Autodesk Inventor part; units mm, degrees
(part 2 of 2)
sketch "Sketch12" plane through (0, 0, 3) normal (0, 0, 1) x (1, 0, 0)
  circle A0 centre (14, 34.5) radius 1.5 projected
  circle A1 centre (-40, -22.5) radius 1.5 projected
  circle A2 centre (-40, 35.5) radius 1.5 projected
  circle A3 centre (46, -22.5) radius 1.5 projected
  circle A4 centre (46, 35.5) radius 1.5 projected
  arc A5 (42.6, 39.5) -> (42, 38.9) centre (42.6, 38.9) ccw projected
  line L0 (42, 38.9) -> (42, 11.25) projected
  arc A6 (40.25, 9.5) -> (42, 11.25) centre (40.25, 11.25) ccw projected
  line L1 (40.25, 9.5) -> (25.75, 9.5) projected
  arc A7 (24, 11.25) -> (25.75, 9.5) centre (25.75, 11.25) ccw projected
  line L2 (24, 11.25) -> (24, 38.9) projected
  arc A8 (24, 38.9) -> (23.4, 39.5) centre (23.4, 38.9) ccw projected
  line L3 (23.4, 39.5) -> (-49.4, 39.5) projected
  arc A9 (-49.4, 39.5) -> (-50, 38.9) centre (-49.4, 38.9) ccw projected
  line L4 (-50, 38.9) -> (-50, 14.5) projected
  line L5 (-78, 14.5) -> (-50, 14.5) projected
  line L6 (-78, -39.5) -> (-78, 14.5) projected
  line L7 (-78, -39.5) -> (49.4, -39.5) projected
  arc A10 (49.4, -39.5) -> (50, -38.9) centre (49.4, -38.9) ccw projected
  line L8 (50, -38.9) -> (50, 38.9) projected
  arc A11 (50, 38.9) -> (49.4, 39.5) centre (49.4, 38.9) ccw projected
  line L9 (49.4, 39.5) -> (42.6, 39.5) projected
  line L10 (-28.5547, -12.5) -> (-27.0547, -12.5) projected
  arc A12 (-25.3047, -14.25) -> (-27.0547, -12.5) centre (-27.0547, -14.25) ccw projected
  line L11 (-25.3047, -14.25) -> (-25.3047, -14.75) projected
  arc A13 (-27.0547, -16.5) -> (-25.3047, -14.75) centre (-27.0547, -14.75) ccw projected
  line L12 (-27.0547, -16.5) -> (-28.5547, -16.5) projected
  arc A14 (-30.3047, -14.75) -> (-28.5547, -16.5) centre (-28.5547, -14.75) ccw projected
  line L13 (-30.3047, -14.75) -> (-30.3047, -14.25) projected
  arc A15 (-28.5547, -12.5) -> (-30.3047, -14.25) centre (-28.5547, -14.25) ccw projected
  line L14 (2.5, -14.25) -> (2.5, -14.75) projected
  arc A16 (0.75, -16.5) -> (2.5, -14.75) centre (0.75, -14.75) ccw projected
  line L15 (0.75, -16.5) -> (-0.75, -16.5) projected
  arc A17 (-2.5, -14.75) -> (-0.75, -16.5) centre (-0.75, -14.75) ccw projected
  line L16 (-2.5, -14.75) -> (-2.5, -14.25) projected
  arc A18 (-0.75, -12.5) -> (-2.5, -14.25) centre (-0.75, -14.25) ccw projected
  line L17 (-0.75, -12.5) -> (0.75, -12.5) projected
  arc A19 (2.5, -14.25) -> (0.75, -12.5) centre (0.75, -14.25) ccw projected
  line L18 (37.5, -14.75) -> (37.5, -14.25) projected
  arc A20 (39.25, -12.5) -> (37.5, -14.25) centre (39.25, -14.25) ccw projected
  line L19 (39.25, -12.5) -> (40.75, -12.5) projected
  arc A21 (42.5, -14.25) -> (40.75, -12.5) centre (40.75, -14.25) ccw projected
  line L20 (42.5, -14.25) -> (42.5, -14.75) projected
  arc A22 (40.75, -16.5) -> (42.5, -14.75) centre (40.75, -14.75) ccw projected
  line L21 (40.75, -16.5) -> (39.25, -16.5) projected
  arc A23 (37.5, -14.75) -> (39.25, -16.5) centre (39.25, -14.75) ccw projected
  line L22 (32.75, -27) -> (33.25, -27) projected
  arc A24 (35, -28.75) -> (33.25, -27) centre (33.25, -28.75) ccw projected
  line L23 (35, -28.75) -> (35, -30.25) projected
  arc A25 (33.25, -32) -> (35, -30.25) centre (33.25, -30.25) ccw projected
  line L24 (33.25, -32) -> (32.75, -32) projected
  arc A26 (31, -30.25) -> (32.75, -32) centre (32.75, -30.25) ccw projected
  line L25 (31, -30.25) -> (31, -28.75) projected
  arc A27 (32.75, -27) -> (31, -28.75) centre (32.75, -28.75) ccw projected
  line L26 (-2.5, 18.75) -> (-2.5, 20.25) projected
  arc A28 (-0.75, 22) -> (-2.5, 20.25) centre (-0.75, 20.25) ccw projected
  line L27 (-0.75, 22) -> (-0.25, 22) projected
  arc A29 (1.5, 20.25) -> (-0.25, 22) centre (-0.25, 20.25) ccw projected
  line L28 (1.5, 20.25) -> (1.5, 18.75) projected
  arc A30 (-0.25, 17) -> (1.5, 18.75) centre (-0.25, 18.75) ccw projected
  line L29 (-0.25, 17) -> (-0.75, 17) projected
  arc A31 (-2.5, 18.75) -> (-0.75, 17) centre (-0.75, 18.75) ccw projected
  line L30 (-30.3047, 5.25) -> (-30.3047, 5.75) projected
  arc A32 (-28.5547, 7.5) -> (-30.3047, 5.75) centre (-28.5547, 5.75) ccw projected
  line L31 (-28.5547, 7.5) -> (-27.0547, 7.5) projected
  arc A33 (-25.3047, 5.75) -> (-27.0547, 7.5) centre (-27.0547, 5.75) ccw projected
  line L32 (-25.3047, 5.75) -> (-25.3047, 5.25) projected
  arc A34 (-27.0547, 3.5) -> (-25.3047, 5.25) centre (-27.0547, 5.25) ccw projected
  line L33 (-27.0547, 3.5) -> (-28.5547, 3.5) projected
  arc A35 (-30.3047, 5.25) -> (-28.5547, 3.5) centre (-28.5547, 5.25) ccw projected
  line L34 (-0.75, -26.5) -> (0.75, -26.5) projected
  arc A36 (2.5, -28.25) -> (0.75, -26.5) centre (0.75, -28.25) ccw projected
  line L35 (2.5, -28.25) -> (2.5, -28.75) projected
  arc A37 (0.75, -30.5) -> (2.5, -28.75) centre (0.75, -28.75) ccw projected
  line L36 (0.75, -30.5) -> (-0.75, -30.5) projected
  arc A38 (-2.5, -28.75) -> (-0.75, -30.5) centre (-0.75, -28.75) ccw projected
  line L37 (-2.5, -28.75) -> (-2.5, -28.25) projected
  arc A39 (-0.75, -26.5) -> (-2.5, -28.25) centre (-0.75, -28.25) ccw projected
  line L38 (39.25, 7.5) -> (40.75, 7.5) projected
  arc A40 (42.5, 5.75) -> (40.75, 7.5) centre (40.75, 5.75) ccw projected
  line L39 (42.5, 5.75) -> (42.5, 5.25) projected
  arc A41 (40.75, 3.5) -> (42.5, 5.25) centre (40.75, 5.25) ccw projected
  line L40 (40.75, 3.5) -> (39.25, 3.5) projected
  arc A42 (37.5, 5.25) -> (39.25, 3.5) centre (39.25, 5.25) ccw projected
  line L41 (37.5, 5.25) -> (37.5, 5.75) projected
  arc A43 (39.25, 7.5) -> (37.5, 5.75) centre (39.25, 5.75) ccw projected
  line L42 (19.25, -32) -> (18.75, -32) projected
  arc A44 (17, -30.25) -> (18.75, -32) centre (18.75, -30.25) ccw projected
  line L43 (17, -30.25) -> (17, -28.75) projected
  arc A45 (18.75, -27) -> (17, -28.75) centre (18.75, -28.75) ccw projected
  line L44 (18.75, -27) -> (19.25, -27) projected
  arc A46 (21, -28.75) -> (19.25, -27) centre (19.25, -28.75) ccw projected
  line L45 (21, -28.75) -> (21, -30.25) projected
  arc A47 (19.25, -32) -> (21, -30.25) centre (19.25, -30.25) ccw projected
  line L46 (-22.5, 18.75) -> (-22.5, 20.25) projected
  arc A48 (-20.75, 22) -> (-22.5, 20.25) centre (-20.75, 20.25) ccw projected
  line L47 (-20.75, 22) -> (-20.25, 22) projected
  arc A49 (-18.5, 20.25) -> (-20.25, 22) centre (-20.25, 20.25) ccw projected
  line L48 (-18.5, 20.25) -> (-18.5, 18.75) projected
  arc A50 (-20.25, 17) -> (-18.5, 18.75) centre (-20.25, 18.75) ccw projected
  line L49 (-20.25, 17) -> (-20.75, 17) projected
  arc A51 (-22.5, 18.75) -> (-20.75, 17) centre (-20.75, 18.75) ccw projected
  line L50 (-24, -34.25) -> (-24, -32.75) projected
  arc A52 (-22.25, -31) -> (-24, -32.75) centre (-22.25, -32.75) ccw projected
  line L51 (-22.25, -31) -> (-21.75, -31) projected
  arc A53 (-20, -32.75) -> (-21.75, -31) centre (-21.75, -32.75) ccw projected
  line L52 (-20, -32.75) -> (-20, -34.25) projected
  arc A54 (-21.75, -36) -> (-20, -34.25) centre (-21.75, -34.25) ccw projected
  line L53 (-21.75, -36) -> (-22.25, -36) projected
  arc A55 (-24, -34.25) -> (-22.25, -36) centre (-22.25, -34.25) ccw projected
  line L54 (40.2277, -23) -> (39.7277, -23) projected
  arc A56 (37.9777, -21.25) -> (39.7277, -23) centre (39.7277, -21.25) ccw projected
  line L55 (37.9777, -21.25) -> (37.9777, -19.75) projected
  arc A57 (39.7277, -18) -> (37.9777, -19.75) centre (39.7277, -19.75) ccw projected
  line L56 (39.7277, -18) -> (40.2277, -18) projected
  arc A58 (41.9777, -19.75) -> (40.2277, -18) centre (40.2277, -19.75) ccw projected
  line L57 (41.9777, -19.75) -> (41.9777, -21.25) projected
  arc A59 (40.2277, -23) -> (41.9777, -21.25) centre (40.2277, -21.25) ccw projected
  line L58 (-33, -34.25) -> (-33, -32.75) projected
  arc A60 (-31.25, -31) -> (-33, -32.75) centre (-31.25, -32.75) ccw projected
  line L59 (-31.25, -31) -> (-30.75, -31) projected
  arc A61 (-29, -32.75) -> (-30.75, -31) centre (-30.75, -32.75) ccw projected
  line L60 (-29, -32.75) -> (-29, -34.25) projected
  arc A62 (-30.75, -36) -> (-29, -34.25) centre (-30.75, -34.25) ccw projected
  line L61 (-30.75, -36) -> (-31.25, -36) projected
  arc A63 (-33, -34.25) -> (-31.25, -36) centre (-31.25, -34.25) ccw projected
  line L62 (28.9777, -21.25) -> (28.9777, -19.75) projected
  arc A64 (30.7277, -18) -> (28.9777, -19.75) centre (30.7277, -19.75) ccw projected
  line L63 (30.7277, -18) -> (31.2277, -18) projected
  arc A65 (32.9777, -19.75) -> (31.2277, -18) centre (31.2277, -19.75) ccw projected
  line L64 (32.9777, -19.75) -> (32.9777, -21.25) projected
  arc A66 (31.2277, -23) -> (32.9777, -21.25) centre (31.2277, -21.25) ccw projected
  line L65 (31.2277, -23) -> (30.7277, -23) projected
  arc A67 (28.9777, -21.25) -> (30.7277, -23) centre (30.7277, -21.25) ccw projected
  line L66 (5.75, 11.5) -> (4.25, 11.5) projected
  arc A68 (2.5, 13.25) -> (4.25, 11.5) centre (4.25, 13.25) ccw projected
  line L67 (2.5, 13.25) -> (2.5, 13.75) projected
  arc A69 (4.25, 15.5) -> (2.5, 13.75) centre (4.25, 13.75) ccw projected
  line L68 (4.25, 15.5) -> (5.75, 15.5) projected
  arc A70 (7.5, 13.75) -> (5.75, 15.5) centre (5.75, 13.75) ccw projected
  line L69 (7.5, 13.75) -> (7.5, 13.25) projected
  arc A71 (5.75, 11.5) -> (7.5, 13.25) centre (5.75, 13.25) ccw projected
  line L70 (-32.5, 7.75) -> (-32.5, 7.25) projected
  arc A72 (-34.25, 5.5) -> (-32.5, 7.25) centre (-34.25, 7.25) ccw projected
  line L71 (-34.25, 5.5) -> (-35.75, 5.5) projected
  arc A73 (-37.5, 7.25) -> (-35.75, 5.5) centre (-35.75, 7.25) ccw projected
  line L72 (-37.5, 7.25) -> (-37.5, 7.75) projected
  arc A74 (-35.75, 9.5) -> (-37.5, 7.75) centre (-35.75, 7.75) ccw projected
  line L73 (-35.75, 9.5) -> (-34.25, 9.5) projected
  arc A75 (-32.5, 7.75) -> (-34.25, 9.5) centre (-34.25, 7.75) ccw projected
  line L74 (7.5, 7.75) -> (7.5, 7.25) projected
  arc A76 (5.75, 5.5) -> (7.5, 7.25) centre (5.75, 7.25) ccw projected
  line L75 (5.75, 5.5) -> (4.25, 5.5) projected
  arc A77 (2.5, 7.25) -> (4.25, 5.5) centre (4.25, 7.25) ccw projected
  line L76 (2.5, 7.25) -> (2.5, 7.75) projected
  arc A78 (4.25, 9.5) -> (2.5, 7.75) centre (4.25, 7.75) ccw projected
  line L77 (4.25, 9.5) -> (5.75, 9.5) projected
  arc A79 (7.5, 7.75) -> (5.75, 9.5) centre (5.75, 7.75) ccw projected
  line L78 (-34.25, 11.5) -> (-35.75, 11.5) projected
  arc A80 (-37.5, 13.25) -> (-35.75, 11.5) centre (-35.75, 13.25) ccw projected
  line L79 (-37.5, 13.25) -> (-37.5, 13.75) projected
  arc A81 (-35.75, 15.5) -> (-37.5, 13.75) centre (-35.75, 13.75) ccw projected
  line L80 (-35.75, 15.5) -> (-34.25, 15.5) projected
  arc A82 (-32.5, 13.75) -> (-34.25, 15.5) centre (-34.25, 13.75) ccw projected
  line L81 (-32.5, 13.75) -> (-32.5, 13.25) projected
  arc A83 (-34.25, 11.5) -> (-32.5, 13.25) centre (-34.25, 13.25) ccw projected
  line L82 (-50, 14.5) -> (-78, 14.5)
  line L83 (-78, 14.5) -> (-78, -18.5)
  line L84 (-78, -18.5) -> (-50, -18.5)
  line L85 (-50, -18.5) -> (-50, 14.5)
  line L86 (-78, -39.5) -> (-78, 14.5) projected
  point P0 (0, 0)
  point P1 (-78, -18.5)
  dimension "d163" = 33
  constraints: 8 end point, 2 parallel, 1 horizontal, 1 perpendicular, 1 point on line
  measures "d163" distance between parallel lines of L5 L84
extrude "Extrusion12" cut sketch "Sketch12" against normal blind 4.6 contours L6 L5 L85 L84
fillet "Fillet7" radius 1.75 1 edges at (-50, -18.5, 0.7)
sketch "Sketch13" plane through (0, 0, -1.6) normal (0, 0, 1) x (1, 0, 0)
  arc A0 (-51.75, -18.5) -> (-50, -16.75) centre (-51.75, -16.75) ccw projected
  line L0 (-50, 14.5) -> (-50, -16.75) projected
  line L1 (-78, 14.5) -> (-50, 14.5) projected
  line L2 (-78, -18.5) -> (-78, 14.5) projected
  line L3 (-51.75, -18.5) -> (-78, -18.5) projected
  line L4 (-64, 14.5) -> (-64, -18.5) construction
  circle A1 centre (-64, 11.325) radius 1.75
  circle A2 centre (-64, -14.075) radius 1.75
  point P0 (0, 0)
  dimension "d169" = 3.5
  dimension "d170" = 3.5
  dimension "d171" = 25.4
  dimension "d172" = 3.175
  constraints: 3 point on line, 2 centre point, 2 end point, 1 midpoint, 1 perpendicular
  measures "d169" diameter of A1
  measures "d170" diameter of A2
  measures "d171" distance of A2.centre A1.centre
  measures "d172" distance from line of L1 A1.centre
extrude "Extrusion13" cut sketch "Sketch13" against normal through all contours A1 | A2
sketch "Sketch14" plane through (0, 0, 3) normal (0, 0, 1) x (1, 0, 0)
  line L0 (-78, -39.5) -> (49.4, -39.5) projected
  line L1 (-78, -39.5) -> (-50, -39.5)
  line L2 (-50, -39.5) -> (-50, -29.5)
  line L3 (-50, -29.5) -> (-78, -29.5)
  line L4 (-78, -29.5) -> (-78, -39.5)
  point P0 (0, 0)
  point P1 (-50, -16.75)
  dimension "d175" = 10
  constraints: 8 end point, 2 parallel, 1 horizontal, 1 perpendicular, 1 point on line
  measures "d175" distance between parallel lines of L0 L3
extrude "Extrusion14" cut sketch "Sketch14" against normal through all
fillet "Fillet8" radius 1.75 1 edges at (-50, -29.5, -0.3)
fillet "Fillet9" radius 0.6 4 edges at (-78, 14.5, -2.6) (-78, -18.5, 0.7) (-78, -29.5, -0.3) (-50, -39.5, -0.3)
sketch "Sketch15" plane through (0, 0, -3.6) normal (0, 0, -1) x (-1, 0, 0)
  line L0 (47, -39.5) -> (78, -39.5)
  line L1 (78, -39.5) -> (78, -20.5)
  line L2 (78, -20.5) -> (47, -20.5)
  line L3 (47, -20.5) -> (47, -39.5)
  line L4 (78, -28.9) -> (78, 13.9) projected
  line L5 (51.75, -18.5) -> (77.4, -18.5) projected
  point P0 (0, 0)
  dimension "d180" = 2
  constraints: 8 end point, 2 parallel, 1 horizontal, 1 perpendicular, 1 point on line
  measures "d180" distance between parallel lines of L5 L2
extrude "Extrusion15" cut sketch "Sketch15" against normal up to surface (3.6 mm away)
fillet "Fillet10" radius 0.6 3 edges at (-47, -20.5, -1.8) (-47, 14.5, -1.8) (-78, -20.5, -1.8)
sketch "Sketch16" plane through (0, 0, 3) normal (0, 0, 1) x (1, 0, 0)
  line L0 (-78, -28.9) -> (-78, -19.1) projected
  line L1 (-73.75, -21) -> (-72.25, -21)
  line L2 (-70.5, -22.75) -> (-70.5, -23.25)
  line L3 (-72.25, -25) -> (-73.75, -25)
  line L4 (-75.5, -23.25) -> (-75.5, -22.75)
  line L5 (-75.5, -21) -> (-70.5, -25) construction
  line L6 (-70.5, -21) -> (-75.5, -25) construction
  arc A0 (-70.5, -22.75) -> (-72.25, -21) centre (-72.25, -22.75) ccw
  arc A1 (-72.25, -25) -> (-70.5, -23.25) centre (-72.25, -23.25) ccw
  arc A2 (-75.5, -23.25) -> (-73.75, -25) centre (-73.75, -23.25) ccw
  arc A3 (-73.75, -21) -> (-75.5, -22.75) centre (-73.75, -22.75) ccw
  line L7 (-77.4, -29.5) -> (-51.75, -29.5) projected
  line L8 (-67.386, -26.25) -> (-82.3219, -26.25) construction
  line L9 (-73.75, -31.5) -> (-72.25, -31.5)
  line L10 (-70.5, -29.75) -> (-70.5, -29.25)
  line L11 (-72.25, -27.5) -> (-73.75, -27.5)
  line L12 (-75.5, -29.25) -> (-75.5, -29.75)
  line L13 (-75.5, -31.5) -> (-70.5, -27.5) construction
  line L14 (-70.5, -31.5) -> (-75.5, -27.5) construction
  arc A4 (-72.25, -31.5) -> (-70.5, -29.75) centre (-72.25, -29.75) ccw
  arc A5 (-70.5, -29.25) -> (-72.25, -27.5) centre (-72.25, -29.25) ccw
  arc A6 (-73.75, -27.5) -> (-75.5, -29.25) centre (-73.75, -29.25) ccw
  arc A7 (-75.5, -29.75) -> (-73.75, -31.5) centre (-73.75, -29.75) ccw
  line L15 (-20.75, 37) -> (-21.25, 37)
  line L16 (-23, 35.25) -> (-23, 33.75)
  line L17 (-21.25, 32) -> (-20.75, 32)
  line L18 (-19, 33.75) -> (-19, 35.25)
  line L19 (-19, 37) -> (-23, 32) construction
  line L20 (-23, 37) -> (-19, 32) construction
  line L21 (-27.25, 37) -> (-27.75, 37)
  line L22 (-29.5, 35.25) -> (-29.5, 33.75)
  line L23 (-27.75, 32) -> (-27.25, 32)
  line L24 (-25.5, 33.75) -> (-25.5, 35.25)
  line L25 (-25.5, 37) -> (-29.5, 32) construction
  line L26 (-29.5, 37) -> (-25.5, 32) construction
  arc A8 (-19, 35.25) -> (-20.75, 37) centre (-20.75, 35.25) ccw
  arc A9 (-20.75, 32) -> (-19, 33.75) centre (-20.75, 33.75) ccw
  arc A10 (-23, 33.75) -> (-21.25, 32) centre (-21.25, 33.75) ccw
  arc A11 (-21.25, 37) -> (-23, 35.25) centre (-21.25, 35.25) ccw
  arc A12 (-25.5, 35.25) -> (-27.25, 37) centre (-27.25, 35.25) ccw
  arc A13 (-27.25, 32) -> (-25.5, 33.75) centre (-27.25, 33.75) ccw
  arc A14 (-29.5, 33.75) -> (-27.75, 32) centre (-27.75, 33.75) ccw
  arc A15 (-27.75, 37) -> (-29.5, 35.25) centre (-27.75, 35.25) ccw
  line L27 (-50, 38.9) -> (-50, -16.75) projected
  line L28 (23.4, 39.5) -> (-49.4, 39.5) projected
  point P0 (0, 0)
  point P1 (-73, -23)
  point P2 (-73, -29.5)
  point P3 (-73, -29.5)
  point P4 (-21, 34.5)
  point P5 (-27.5, 34.5)
  dimension "d187" = 1.75
  dimension "d188" = 1.5
  dimension "d189" = 0.5
  dimension "d190" = 5
  dimension "d196" = 2.5
  dimension "d197" = 2.5
  dimension "d198" = 1.75
  dimension "d199" = 0.5
  dimension "d200" = 0.5
  dimension "d201" = 1.5
  dimension "d202" = 1.5
  dimension "d203" = 22.5
  dimension "d204" = 5
  constraints: 50 end point, 34 point on line, 32 point on circle, 24 tangent, 17 symmetric about line, 16 centre point, 10 equal radius, 7 midpoint, 6 parallel, 4 horizontal, 3 perpendicular, 4 other
  measures "d187" radius of A0
  measures "d188" distance of L3.start L3.end
  measures "d189" distance of L2.start L2.end
  measures "d190" distance from line of L0 point (-73, -23)
  measures "d196" distance between parallel lines of L11 L3
  measures "d197" distance between parallel lines of L16 L24
  measures "d198" radius of A8
  measures "d199" distance of L17.start L17.end
  measures "d200" distance of L23.start L23.end
  measures "d201" distance of L24.start L24.end
  measures "d202" distance of L18.start L18.end
  measures "d203" distance from line of L27 point (-27.5, 34.5)
  measures "d204" distance from line of L28 point (-21, 34.5)
extrude "Extrusion16" cut sketch "Sketch16" against normal through all
fillet "Fillet11" radius 0.6 2 edges at (-70.5, -29.5, 1.5) (-75.5, -29.5, 1.5)
chamfer "Chamfer1" distance 0.5 angle 45 198 edges at (-50, 11.075, 3) (-50.5126, -17.9874, 3) (-64.575, -18.5, 3) (-77.8243, -18.6757, 3) (-78, -24, 3) (-77.8243, -29.3243, 3) (-76.7369, -29.5, 3) (-75.6824, -29.3548, 3) (-74.8916, -27.9236, 3) (-73, -27.5, 3) (-71.1084, -27.9236, 3) (-70.3176, -29.3548, 3) (-60.8381, -29.5, 3) (-50.5126, -30.0126, 3) (-50, -35.075, 3) (-49.8243, -39.3243, 3) (0, -39.5, 3) (49.8243, -39.3243, 3) (50, 0, 3) (49.8243, 39.3243, 3) (46, 39.5, 3) (42.1757, 39.3243, 3) (42, 25.075, 3) (41.4874, 10.0126, 3) (33, 9.5, 3) (24.5126, 10.0126, 3) (24, 25.075, 3) (23.8243, 39.3243, 3) (-13, 39.5, 3) (-49.8243, 39.3243, 3) (-19.0126, 21.4874, 3) (-20.5, 22, 3) (-21.9874, 21.4874, 3) (-22.5, 19.5, 3) (-21.9874, 17.5126, 3) (-20.5, 17, 3) (-19.0126, 17.5126, 3) (-18.5, 19.5, 3) (-33.0126, 14.9874, 3) (-35, 15.5, 3) (-36.9874, 14.9874, 3) (-37.5, 13.5, 3) (-36.9874, 12.0126, 3) (-35, 11.5, 3) (-33.0126, 12.0126, 3) (-32.5, 13.5, 3) (-25.8172, 6.9874, 3) (-27.8047, 7.5, 3) (-29.7921, 6.9874, 3) (-30.3047, 5.5, 3) (-29.7921, 4.0126, 3) (-27.8047, 3.5, 3) (-25.8172, 4.0126, 3) (-25.3047, 5.5, 3) (-33.0126, 8.9874, 3) (-35, 9.5, 3) (-36.9874, 8.9874, 3) (-37.5, 7.5, 3) (-36.9874, 6.0126, 3) (-35, 5.5, 3) (-33.0126, 6.0126, 3) (-32.5, 7.5, 3) (-27.8047, -12.5, 3) (-25.8172, -13.0126, 3) (-25.3047, -14.5, 3) (-25.8172, -15.9874, 3) (-27.8047, -16.5, 3) (-29.7921, -15.9874, 3) (-30.3047, -14.5, 3) (-29.7921, -13.0126, 3) (-29.5126, -31.5126, 3) (-31, -31, 3) (-32.4874, -31.5126, 3) (-33, -33.5, 3) (-32.4874, -35.4874, 3) (-31, -36, 3) (-29.5126, -35.4874, 3) (-29, -33.5, 3) (-20.5126, -31.5126, 3) (-22, -31, 3) (-23.4874, -31.5126, 3) (-24, -33.5, 3) (-23.4874, -35.4874, 3) (-22, -36, 3) (-20.5126, -35.4874, 3) (-20, -33.5, 3) (0, -26.5, 3) (1.9874, -27.0126, 3) (2.5, -28.5, 3) (1.9874, -29.9874, 3) (0, -30.5, 3) (-1.9874, -29.9874, 3) (-2.5, -28.5, 3) (-1.9874, -27.0126, 3) (1.9874, -13.0126, 3) (0, -12.5, 3) (-1.9874, -13.0126, 3) (-2.5, -14.5, 3) (-1.9874, -15.9874, 3) (0, -16.5, 3) (1.9874, -15.9874, 3) (2.5, -14.5, 3) (17.5126, -27.5126, 3) (17, -29.5, 3) (17.5126, -31.4874, 3) (19, -32, 3) (20.4874, -31.4874, 3) (21, -29.5, 3) (20.4874, -27.5126, 3) (19, -27, 3) (34.4874, -27.5126, 3) (33, -27, 3) (31.5126, -27.5126, 3) (31, -29.5, 3) (31.5126, -31.4874, 3) (33, -32, 3) (34.4874, -31.4874, 3) (35, -29.5, 3) (32.4652, -18.5126, 3) (30.9777, -18, 3) (29.4903, -18.5126, 3) (28.9777, -20.5, 3) (29.4903, -22.4874, 3) (30.9777, -23, 3) (32.4652, -22.4874, 3) (32.9777, -20.5, 3) (41.9874, -13.0126, 3) (40, -12.5, 3) (38.0126, -13.0126, 3) (37.5, -14.5, 3) (38.0126, -15.9874, 3) (40, -16.5, 3) (41.9874, -15.9874, 3) (42.5, -14.5, 3) (41.4652, -18.5126, 3) (39.9777, -18, 3) (38.4903, -18.5126, 3) (37.9777, -20.5, 3) (38.4903, -22.4874, 3) (39.9777, -23, 3) (41.4652, -22.4874, 3) (41.9777, -20.5, 3) (41.9874, 6.9874, 3) (40, 7.5, 3) (38.0126, 6.9874, 3) (37.5, 5.5, 3) (38.0126, 4.0126, 3) (40, 3.5, 3) (41.9874, 4.0126, 3) (42.5, 5.5, 3) (6.9874, 8.9874, 3) (5, 9.5, 3) (3.0126, 8.9874, 3) (2.5, 7.5, 3) (3.0126, 6.0126, 3) (5, 5.5, 3) (6.9874, 6.0126, 3) (7.5, 7.5, 3) (6.9874, 14.9874, 3) (5, 15.5, 3) (3.0126, 14.9874, 3) (2.5, 13.5, 3) (3.0126, 12.0126, 3) (5, 11.5, 3) (6.9874, 12.0126, 3) (7.5, 13.5, 3) (0.9874, 21.4874, 3) (-0.5, 22, 3) (-1.9874, 21.4874, 3) (-2.5, 19.5, 3) (-1.9874, 17.5126, 3) (-0.5, 17, 3) (0.9874, 17.5126, 3) (1.5, 19.5, 3) (-71.0126, -21.5126, 3) (-70.5, -23, 3) (-71.0126, -24.4874, 3) (-73, -25, 3) (-74.9874, -24.4874, 3) (-75.5, -23, 3) (-74.9874, -21.5126, 3) (-73, -21, 3) (-25.5, 34.5, 3) (-26.0126, 32.5126, 3) (-27.5, 32, 3) (-28.9874, 32.5126, 3) (-29.5, 34.5, 3) (-28.9874, 36.4874, 3) (-27.5, 37, 3) (-26.0126, 36.4874, 3) (-21, 32, 3) (-22.4874, 32.5126, 3) (-23, 34.5, 3) (-22.4874, 36.4874, 3) (-21, 37, 3) (-19.5126, 36.4874, 3) (-19, 34.5, 3) (-19.5126, 32.5126, 3)
equation "\"d5\" = d4"
equation "\"d8\" = d7"
equation "\"d21\" = d14"
equation "\"d25\" = d24"
equation "\"d26\" = d24"
equation "\"d27\" = d26"
equation "\"d29\" = d26"
equation "\"d30\" = d26"
equation "\"d31\" = d24"
equation "\"d32\" = d24"
equation "\"d33\" = d24"
equation "\"d38\" = d37"
equation "\"d46\" = d29"
equation "\"d47\" = d36"
equation "\"d56\" = d54"
equation "\"d57\" = d55"
equation "\"d61\" = d63"
equation "\"d73\" = d79"
equation "\"d75\" = d81"
equation "\"d89\" = d88"
equation "\"d90\" = d89"
equation "\"d91\" = d87"
equation "\"d92\" = d91"
equation "\"d107\" = d117"
equation "\"d108\" = d107"
equation "\"d63\" = 5"
equation "\"d79\" = 5"
equation "\"d81\" = 5"
equation "\"d117\" = 5"
body "Solid1"
